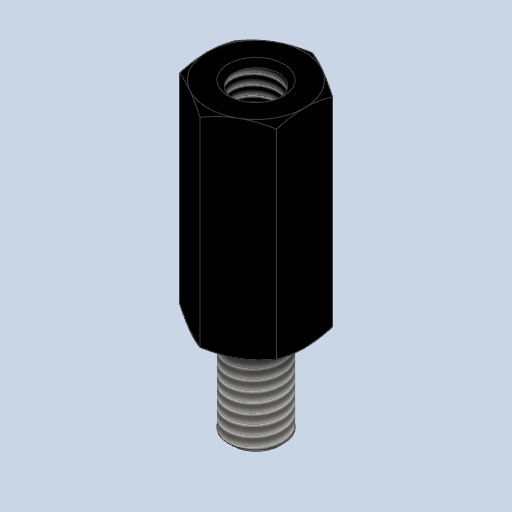
# Autodesk Inventor part: BSL-415BE
Saved by Autodesk Inventor 2022 (Build 260153000, 153)
## iProperties
Part Number: BSL-415BE
Material: アルミニウム 2014-T4
Document SubType Name: Modeling
Designer: Masato Kubotera
Density: 3.71165 g/cm^3
Appearance: 黒
Catalog Web Link: https://www.hirosugi-net.co.jp/shop/g/g13345/
Description: ReadyMade
Mass: 0.723 g
Surface Area: 6.11044 cm^2
Volume: 0.653703 cm^3
Author: Masato Kubotera
Comments: Width across flats : 7.0
Autodesk Inventor part; units mm, degrees
ref_plane "YZ Plane" through (0, 0, 0) normal (1, 0, 0) x (0, 1, 0)
ref_plane "XZ Plane" through (0, 0, 0) normal (0, 1, 0) x (-1, 0, 0)
ref_plane "XY Plane" through (0, 0, 0) normal (0, 0, 1) x (1, 0, 0)
sketch "スケッチ1" plane through (0, 0, 0) normal (1, 0, 0) x (0, 1, 0)
  line L0 (-7.5, 0) -> (7.5, 0)
  line L1 (0, 0) -> (0, 4.0415) construction
  line L2 (-7.1874, 4.0415) -> (-7.5, 3.5)
  line L3 (-7.5, 3.5) -> (-7.5, 0)
  line L4 (-7.1874, 4.0415) -> (7.1874, 4.0415)
  line L5 (7.1874, 4.0415) -> (7.5, 3.5)
  line L6 (7.5, 3.5) -> (7.5, 0)
  line L7 (-7.5, 2) -> (-14.2, 2)
  line L8 (-14.5, 1.7) -> (-14.5, 0)
  line L9 (-14.5, 0) -> (-7.5, 0)
  line L10 (-14.2, 2) -> (-14.5, 1.7)
  point P0 (7.5, 1.5)
  point P1 (-14.5, 2)
  dimension "d1" = 3.5
  dimension "d2" = 4.0415
  dimension "d3" = 30
  dimension "d4" = 15
  dimension "d18" = 7
  dimension "d19" = 4
  dimension "d22" = 0.3
  dimension "d23" = 0.3
  constraints: 22 end point, 4 perpendicular, 4 point on line, 2 horizontal, 2 midpoint, 1 coincident, 1 collinear, 1 symmetric about line
  measures "d1" distance of L0.start L2.end
  measures "d2" vertical distance of L0.start L2.start
  measures "d3" angle of L3 L2
  measures "d4" distance of L0.start L0.end
  measures "d18" distance of L7.start point (-14.5, 2)
  measures "d19" diameter of L7 L9
  measures "d22" distance of L7.end point (-14.5, 2)
  measures "d23" distance of L8.start point (-14.5, 2)
revolve "回転1" add sketch "スケッチ1" angle 360 about axis through (0, -7.5, 0) along (0, 1, 0)
sketch "スケッチ2" plane through (0, 7.5, 0) normal (0, 1, 0) x (1, 0, 0)
  line L0 (0, -4.0415) -> (-3.5, -2.0207)
  line L1 (-3.5, -2.0207) -> (-3.5, 2.0207)
  line L2 (-3.5, 2.0207) -> (0, 4.0415)
  line L3 (0, 4.0415) -> (3.5, 2.0207)
  line L4 (3.5, 2.0207) -> (3.5, -2.0207)
  line L5 (3.5, -2.0207) -> (0, -4.0415)
  circle A0 centre (0, 0) radius 4.0415 projected
  point P0 (0, 0)
  point P1 (0, 0)
  point P2 (3.5, 2.0207)
  point P3 (3.5, 2.0207)
  point P4 (0, 4.0415)
  point P5 (0, 4.0415)
  point P6 (-3.5, 2.0207)
  point P7 (-3.5, 2.0207)
  point P8 (-3.5, -2.0207)
  point P9 (3.5, -2.0207)
  point P10 (3.5, -2.0207)
  constraints: 12 end point, 2 coincident, 1 vertical, 15 other
extrude "押し出し1" cut sketch "スケッチ2" against normal through all contours A0 L0 | L5 A0 | A0 L1 | L4 A0 | A0 L2 | L3 A0
hole "穴1" at (0, 7.5, 0) direction (0, -1, 0) diameter 3.242 depth 8 tip angle 118 countersink diameter 4 countersink angle 90 thread size "M4x0.7" class "6H" standard "ISO Metric profile"
thread "ねじ1" size "M4x0.7" class "6g" standard "ANSI Metric M Profile" full length
equation "\"d2\" = 1.1547 * d1"
equation "\"d23\" = d22"
